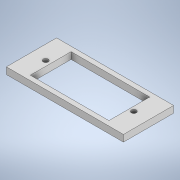
# Autodesk Inventor part: servo housing lid
Saved by Autodesk Inventor 2022 (Build 260153000, 153)
## iProperties
Created: 2022-01-29
Part Number: servo housing lid
Material: Generic
Document SubType Name: Modeling
Designer: peter
Density: 1 g/cm^3
Appearance: Default
Author: peter
Autodesk Inventor part; units mm, degrees
ref_plane "YZ Plane" through (0, 0, 0) normal (1, 0, 0) x (0, 1, 0)
ref_plane "XZ Plane" through (0, 0, 0) normal (0, 1, 0) x (-1, 0, 0)
ref_plane "XY Plane" through (0, 0, 0) normal (0, 0, 1) x (1, 0, 0)
sketch "Sketch1" plane through (0, 0, 0) normal (0, 1, 0) x (-1, 0, 0)
  line L0 (17.5, -7.5) -> (-17.5, -7.5)
  line L1 (-17.5, -7.5) -> (-17.5, 7.5)
  line L2 (-17.5, 7.5) -> (17.5, 7.5)
  line L3 (17.5, 7.5) -> (17.5, -7.5)
  line L4 (17.5, -7.5) -> (-17.5, 7.5) construction
  line L5 (-17.5, -7.5) -> (17.5, 7.5) construction
  line L6 (11.75, -6.1) -> (-11.75, -6.1)
  line L7 (-11.75, -6.1) -> (-11.75, 6.1)
  line L8 (-11.75, 6.1) -> (11.75, 6.1)
  line L9 (11.75, 6.1) -> (11.75, -6.1)
  line L10 (11.75, -6.1) -> (-11.75, 6.1) construction
  line L11 (-11.75, -6.1) -> (11.75, 6.1) construction
  circle A0 centre (13.25, 0) radius 0.75
  circle A1 centre (-13.1, 0) radius 0.75
  point P0 (0, 0)
  dimension "d37" = 35
  dimension "d38" = 15
  dimension "d39" = 5.75
  dimension "d40" = 5.75
  dimension "d41" = 12.2
  dimension "d42" = 1.5
  dimension "d43" = 1.5
  dimension "d44" = 4.25
  dimension "d45" = 5.15
  constraints: 24 end point, 4 midpoint, 3 parallel, 2 centre point, 2 horizontal, 1 perpendicular
  measures "d37" distance of L0.start L0.end
  measures "d38" distance of L2.end L0.start
  measures "d39" distance between parallel lines of L3 L9
  measures "d40" distance between parallel lines of L1 L7
  measures "d41" distance of L8.end L6.start
  measures "d42" diameter of A0
  measures "d43" diameter of A1
  measures "d44" distance from line of L3 A0.centre
extrude "Extrusion4" add sketch "Sketch1" along normal blind 2
body "Solid2"
